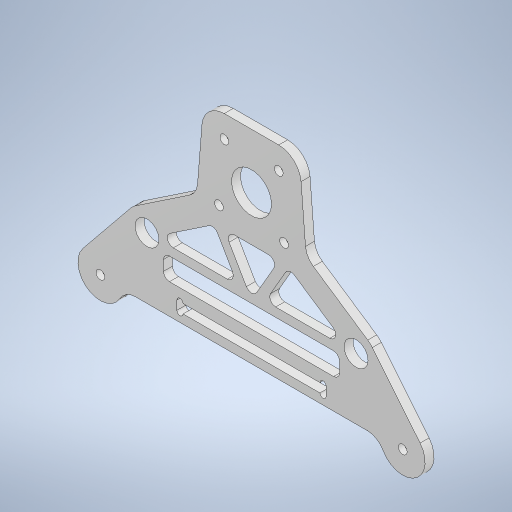
# Autodesk Inventor part: 中間ユニット内
Saved by Autodesk Inventor 2023 (Build 270158000, 158)
## iProperties
Created: 2022-03-07
Part Number: 中間ユニット内
Material: Aluminum 2014-T6
Document SubType Name: Modeling
Designer: acps
Density: 2.78927 g/cm^3
Appearance: Satin
Author: acps
Autodesk Inventor part; units mm, degrees
ref_plane "YZ Plane" through (0, 0, 0) normal (1, 0, 0) x (0, 1, 0)
ref_plane "XZ Plane" through (0, 0, 0) normal (0, 1, 0) x (-1, 0, 0)
ref_plane "XY Plane" through (0, 0, 0) normal (0, 0, 1) x (1, 0, 0)
sketch "Sketch2" plane through (0, 0, 0) normal (0, 0, 1) x (1, 0, 0)
  line L0 (0, 0) -> (0, 5.2095) construction
  circle A0 centre (0, 29.1078) radius 6.7008
  arc A1 (-5.7731, 13.9993) -> (-7.5051, 10.9993) centre (-5.7731, 11.9993) ccw
  line L1 (-5.7731, 13.9993) -> (5.7731, 13.9993)
  arc A2 (7.5051, 10.9993) -> (5.7731, 13.9993) centre (5.7731, 11.9993) ccw
  line L2 (-7.5051, 10.9993) -> (-1.7321, 1)
  line L3 (7.5051, 10.9993) -> (1.7321, 1)
  arc A3 (-1.7321, 1) -> (1.7321, 1) centre (0, 2) ccw
  line L4 (-25, -16) -> (25, -16) construction
  line L5 (-23.95, -14.5) -> (-23.95, -17.5) construction
  line L6 (-25, -14.5) -> (-25, -17.5)
  line L7 (-22.9, -17.5) -> (-22.9, -14.5) construction
  arc A4 (-22.9, -14.5) -> (-25, -14.5) centre (-23.95, -14.5) ccw
  arc A5 (-25, -17.5) -> (-22.9, -17.5) centre (-23.95, -17.5) ccw
  arc A6 (25, -14.5) -> (22.9, -14.5) centre (23.95, -14.5) ccw
  line L8 (25, -14.5) -> (25, -17.5)
  arc A7 (22.9, -17.5) -> (25, -17.5) centre (23.95, -17.5) ccw
  line L9 (14.2621, 12.4306) -> (27.3148, 3.6601)
  arc A8 (26.1994, 0) -> (27.3148, 3.6601) centre (26.1994, 2) ccw
  line L10 (26.1994, 0) -> (8.0829, 0)
  line L11 (-25, -14.5) -> (-23.95, -14.5) construction
  line L12 (-22.9, -14.5) -> (22.9, -14.5)
  line L13 (-25, -17.5) -> (-23.95, -17.5) construction
  line L14 (-22.9, -17.5) -> (22.9, -17.5)
  line L15 (-27.4866, -3) -> (27.4866, -3)
  line L16 (29.4866, -5) -> (29.4866, -8.45)
  arc A9 (29.4866, -5) -> (27.4866, -3) centre (27.4866, -5) ccw
  line L17 (-26.5636, -13.45) -> (-22.5758, -13.45) construction
  line L18 (-27.4866, -10.45) -> (27.4866, -10.45)
  arc A10 (27.4866, -10.45) -> (29.4866, -8.45) centre (27.4866, -8.45) ccw
  circle A11 centre (9.1116, 40) radius 4.5
  circle A12 centre (9.1116, 40) radius 1.5
  circle A13 centre (10.8954, 20) radius 4.5
  circle A14 centre (10.8954, 20) radius 1.5
  circle A15 centre (35, 0) radius 7.025
  circle A16 centre (35, 0) radius 4.025
  circle A17 centre (50.6355, -20) radius 4.5
  circle A18 centre (50.6355, -20) radius 1.5
  line L19 (38.8033, -20.5) -> (0, -20.5)
  circle A19 centre (-9.1116, 40) radius 4.5
  circle A20 centre (-9.1116, 40) radius 1.5
  circle A21 centre (-10.8954, 20) radius 4.5
  circle A22 centre (-10.8954, 20) radius 1.5
  line L20 (-14.2621, 12.4306) -> (-27.3148, 3.6601)
  line L21 (-26.1994, 0) -> (-8.0829, 0)
  arc A23 (-27.3148, 3.6601) -> (-26.1994, 0) centre (-26.1994, 2) ccw
  circle A24 centre (-35, 0) radius 7.025
  circle A25 centre (-35, 0) radius 4.025
  line L22 (-38.8033, -20.5) -> (0, -20.5)
  arc A26 (-27.4866, -3) -> (-29.4866, -5) centre (-27.4866, -5) ccw
  line L23 (-29.4866, -5) -> (-29.4866, -8.45)
  arc A27 (-29.4866, -8.45) -> (-27.4866, -10.45) centre (-27.4866, -8.45) ccw
  arc A28 (14.2621, 12.4306) -> (11.4146, 11.7706) centre (13.1466, 10.7706) ccw
  line L24 (11.4146, 11.7706) -> (6.3509, 3)
  arc A29 (6.3509, 3) -> (8.0829, 0) centre (8.0829, 2) ccw
  arc A30 (-11.4146, 11.7706) -> (-14.2621, 12.4306) centre (-13.1466, 10.7706) ccw
  line L25 (-11.4146, 11.7706) -> (-6.3509, 3)
  arc A31 (-8.0829, 0) -> (-6.3509, 3) centre (-8.0829, 2) ccw
  circle A32 centre (10.8954, 20) radius 7.5
  circle A33 centre (9.1116, 40) radius 7.5
  line L26 (16.5866, 40.6126) -> (18.0657, 22.5628)
  arc A34 (18.0657, 22.5628) -> (20.6993, 18.0726) centre (24.0457, 23.0528) ccw
  line L27 (20.6993, 18.0726) -> (38.918, 5.8309)
  circle A35 centre (50.6355, -20) radius 7.5
  line L28 (40.4525, 4.4295) -> (56.4567, -15.271)
  arc A36 (44.0621, -23.6111) -> (38.8033, -20.5) centre (38.8033, -26.5) ccw
  line L29 (9.1116, 47.5) -> (0, 47.5)
  line L30 (-9.1116, 47.5) -> (0, 47.5)
  circle A37 centre (-9.1116, 40) radius 7.5
  line L31 (-16.5866, 40.6126) -> (-18.0657, 22.5628)
  line L32 (-20.6993, 18.0726) -> (-38.918, 5.8309)
  circle A38 centre (-10.8954, 20) radius 7.5
  line L33 (-40.4525, 4.4295) -> (-56.4567, -15.271)
  circle A39 centre (-50.6355, -20) radius 7.5
  line L34 (-38.8033, -20.5) -> (0, -20.5)
  arc A40 (-38.8033, -20.5) -> (-44.0621, -23.6111) centre (-38.8033, -26.5) ccw
  circle A41 centre (-50.6355, -20) radius 4.5
  circle A42 centre (-50.6355, -20) radius 1.5
  arc A43 (-20.6993, 18.0726) -> (-18.0657, 22.5628) centre (-24.0457, 23.0528) ccw
  point P0 (-23.95, -16)
  point P1 (0, 0)
  point P2 (-38.918, 5.8309)
  dimension "d164" = 2
  dimension "d165" = 2
  dimension "d166" = 30
  dimension "d167" = 2
  dimension "d168" = 50
  dimension "d169" = 3
  dimension "d170" = 2.1
  dimension "d171" = 25
  dimension "d172" = 2
  dimension "d173" = 3
  dimension "d174" = 2
  dimension "d175" = 3
  dimension "d176" = 7.45
  dimension "d177" = 2
  dimension "d178" = 60
  dimension "d179" = 3
  dimension "d180" = 2
  dimension "d181" = 2
  dimension "d182" = 3
  dimension "d183" = 3
  dimension "d184" = 3
  dimension "d185" = 6
  dimension "d186" = 3
  dimension "d187" = 6
  constraints: 72 end point, 54 point on circle, 44 centre point, 41 symmetric about line, 37 tangent, 7 horizontal, 7 parallel, 3 midpoint, 3 vertical, 2 point on line, 1 horizontal alignment, 1 vertical alignment, 31 other
  measures "d164" radius of A2
  measures "d165" radius of A3
  measures "d166" angle of L0 L2
  measures "d167" radius of A1
  measures "d168" distance of L4.start L4.end
  measures "d169" distance of L5.start L5.end
  measures "d170" diameter of A5
  measures "d171" horizontal distance of point (-25, -16) L0.start
  measures "d172" radius of A9
  measures "d173" distance between parallel lines of L17 L18
  measures "d174" radius of A10
  measures "d175" distance between parallel lines of L15 L10
  measures "d176" distance between parallel lines of L18 L15
  measures "d177" radius of A8
  measures "d178" angle of L2 L3
  measures "d179" distance between parallel lines of L19 L14
  measures "d180" radius of A28
  measures "d181" radius of A29
  measures "d182" distance between parallel lines of L3 L24
  measures "d183" radial gap between concentric circles of A13 A32
  measures "d184" radial gap between concentric circles of A11 A33
  measures "d185" radius of A34
  measures "d186" radial gap between concentric circles of A17 A35
  measures "d187" radius of A36
extrude "Extrusion1" add sketch "Sketch2" against normal blind 3 contours A0 A33 L26 A34 A32 | A0 A37 L30 L29 A33 | A33 | A32 A2 L1 A1 A38 A0 | A32 | A0 A38 A43 L31 A37 | A37 | A38 | A34 L27 A15 A8 L9 A28 A32 | A32 A28 L24 A29 L10 A8 A15 A9 L15 A26 A24 A23 L21 A31 L25 A30 A38 A1 L2 A3 L3 A2 | A38 A30 L20 A23 A24 L32 A43 | A15 | A24 | L28 A35 A36 L19 L22 A40 A39 L33 A24 A26 L23 A27 L18 A10 L16 A9 A15 | A35 | A39
extrude "Extrusion2" add sketch "Sketch2" against normal blind 2 contours A11 | A13 | A17 | A19 | A21 | A41
body "Solid1"
